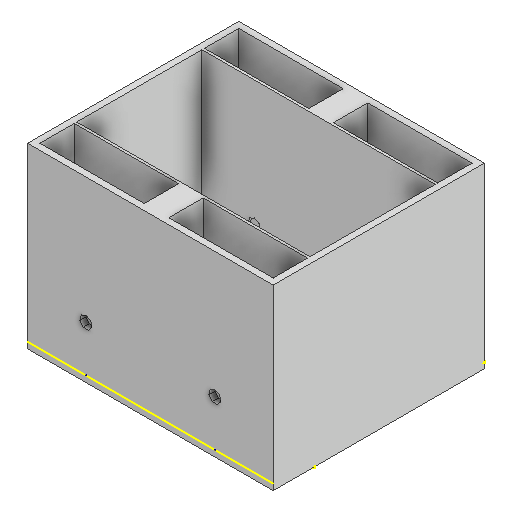
# Autodesk Inventor part: Part2
Saved by Autodesk Inventor 2026.2 (Build 302298010, 298A)
## iProperties
Created: 2026-05-07
Part Number: Part2
Material: Generic
Document SubType Name: Modeling
Designer: danie
Density: 1 g/cm^3
Appearance: Default
Author: danie
Autodesk Inventor part; units mm, degrees
ref_plane "YZ Plane" through (0, 0, 0) normal (1, 0, 0) x (0, 1, 0)
ref_plane "XZ Plane" through (0, 0, 0) normal (0, 1, 0) x (-1, 0, 0)
ref_plane "XY Plane" through (0, 0, 0) normal (0, 0, 1) x (1, 0, 0)
sketch "Sketch1" plane through (0, 0, 0) normal (0, 1, 0) x (-1, 0, 0)
  line L0 (0, 0) -> (200, 0)
  line L1 (200, 0) -> (200, 172)
  line L2 (200, 172) -> (0, 172)
  line L3 (0, 172) -> (0, 0)
  line L4 (0, 172) -> (200, 172)
  line L5 (200, 172) -> (200, -28)
  line L6 (200, -28) -> (0, -28)
  line L7 (0, -28) -> (0, 172)
  line L8 (200, 172) -> (195, 172)
  line L9 (195, 172) -> (195, 167)
  line L10 (195, 167) -> (200, 167)
  line L11 (195, 172) -> (195, 144)
  line L12 (195, 167) -> (130, 167)
  line L13 (130, 167) -> (130, 144)
  line L14 (130, 144) -> (195, 144)
  line L15 (195, 144) -> (195, 0)
  line L16 (195, 0) -> (195, 5)
  line L17 (195, 5) -> (130, 5)
  line L18 (130, 5) -> (130, 33)
  line L19 (130, 33) -> (195, 33)
  line L20 (0, 167) -> (5, 167)
  line L21 (5, 167) -> (5, 139)
  line L22 (130, 167) -> (130, 139)
  line L23 (130, 139) -> (195, 139)
  line L24 (5, 139) -> (70, 139)
  line L25 (70, 139) -> (70, 167)
  line L26 (70, 167) -> (5, 167)
  line L27 (5, 139) -> (5, 0)
  line L28 (5, 33) -> (70, 33)
  line L29 (70, 33) -> (70, 5)
  line L30 (70, 5) -> (5, 5)
  line L31 (130, 139) -> (70, 139)
  line L32 (130, 33) -> (70, 33)
  line L33 (130, 167) -> (70, 167)
  line L34 (130, 5) -> (70, 5)
  line L35 (37.5, 33) -> (37.5, 139)
  line L36 (162.5, 33) -> (162.5, 139)
  line L37 (5, 33) -> (7, 33)
  line L38 (5, 33) -> (5, 35)
  line L39 (5, 35) -> (195, 35)
  line L40 (195, 139) -> (197, 139)
  line L41 (5, 139) -> (5, 137)
  line L42 (5, 137) -> (195, 137)
  line L43 (100, 5) -> (90, 5)
  line L44 (90, 5) -> (110, 5)
  line L45 (110, 5) -> (110, 33)
  line L46 (90, 5) -> (90, 33)
  line L47 (90, 139) -> (90, 167)
  line L48 (110, 137) -> (110, 167)
  point P0 (110, 139)
  dimension "d0" = 200
  dimension "d1" = 172
  dimension "d2" = 200
  dimension "d3" = 200
  dimension "d4" = 5
  dimension "d5" = 5
  dimension "d6" = 28
  dimension "d7" = 65
  dimension "d8" = 5
  dimension "d9" = 28
  dimension "d10" = 5
  dimension "d11" = 28
  dimension "d12" = 28
  dimension "d13" = 65
  dimension "d14" = 2
  dimension "d15" = 2
  dimension "d16" = 2
  dimension "d17" = 2
  dimension "d18" = 10
  dimension "d19" = 20
  constraints: 98 end point, 36 point on line, 20 perpendicular, 6 parallel, 5 midpoint, 3 horizontal, 1 collinear
  measures "d0" distance of L2.end L1.end
  measures "d1" distance of L1.end L0.end
  measures "d2" distance of L5.end L6.end
  measures "d3" distance of L4.end L5.end
  measures "d4" distance of L4.end L8.end
  measures "d5" distance of L8.end L9.end
  measures "d6" distance of L8.end L11.end
  measures "d7" distance of L9.end L12.end
  measures "d8" distance of L15.end L16.end
  measures "d9" distance of L17.end L18.end
  measures "d10" distance of L20.start L20.end
  measures "d11" distance of L20.end L21.end
  measures "d12" distance of L12.end L22.end
  measures "d13" distance of L21.end L24.end
  measures "d14" distance of L28.start L37.end
  measures "d15" distance of L28.start L38.end
  measures "d16" distance of L23.end L40.end
  measures "d17" distance of L21.end L41.end
  measures "d18" distance of L43.start L43.end
  measures "d19" distance of L43.end L44.end
extrude "Extrusion1" add sketch "Sketch1" along normal blind 145 contours L3 L20 L21 L27 L0 | L27 L30 L34 L17 L15 L0 | L3 L2 L9 L12 L33 L26 L20 | L15 L11 L10 L1 L0 | L27 L39 L35 L28 | L2 L1 L10 L9 | L24 L35 L42 L27 | L19 L36 L39 L15 | L28 L35 L39 L36 L19 L32 | L46 L32 L45 L34 | L24 L31 L48 L42 L35 | L33 L48 L31 L47 | L42 L36 L23 L15 | L48 L31 L23 L36 L42
sketch "Sketch2" plane through (0, 0, 0) normal (0, -1, 0) x (1, 0, 0)
  line L0 (-5, 137) -> (-195, 137) projected
  line L1 (-195, 35) -> (-5, 35) projected
  line L2 (-195, 137) -> (-5, 137)
  line L3 (-5, 137) -> (-5, 35)
  line L4 (-5, 35) -> (-195, 35)
  line L5 (-195, 35) -> (-195, 137)
  point P0 (0, 0)
  constraints: 8 end point, 2 parallel, 1 horizontal, 1 perpendicular
extrude "Extrusion2" add sketch "Sketch2" against normal blind 5
sketch "Sketch3" plane through (-195, 0, 139) normal (0, 0, 1) x (1, 0, 0)
  point P0 (195, 0)
sketch "Sketch4" plane through (0, 5, 0) normal (0, 1, 0) x (1, 0, 0)
  line L0 (-90, -33) -> (-90, -5) projected
  line L1 (-5, -33) -> (-90, -33) projected
  line L2 (-90, -33) -> (-5, -33)
  line L3 (-5, -33) -> (-47.5, -33)
  line L4 (-47.5, -33) -> (-47.5, -172)
  line L5 (-200, -172) -> (0, -172) projected
  line L6 (-109.747, -33) -> (-194.7552, -33)
  line L7 (-194.7552, -33) -> (-109.747, -33)
  line L8 (-110, -5) -> (-110, -33) projected
  line L9 (-195, -5) -> (-110, -5) projected
  line L10 (-110, -5) -> (-195, -5)
  line L11 (-195, -5) -> (-152.5, -5)
  line L12 (-152.5, -5) -> (-152.5, -172)
  line L13 (-110, -167) -> (-195, -167) projected
  point P0 (0, 0)
  constraints: 16 end point, 3 collinear, 3 point on line, 2 midpoint, 2 perpendicular
sketch "Sketch5" plane through (-200, 0, 172) normal (0, 0, 1) x (1, 0, 0)
  line L0 (5, 144.4425) -> (89.9982, 145)
  line L1 (0, 145) -> (200, 145) projected
  line L2 (5, 144.4425) -> (47.1963, 145)
  line L3 (47.4991, 144.7212) -> (47.4991, 0)
  line L4 (0, 0) -> (200, 0) projected
  line L5 (200, 145) -> (195, 145)
  line L6 (195, 145) -> (110, 145)
  line L7 (110, 145) -> (152.5, 145)
  line L8 (152.5, 145) -> (152.5, 0)
  line L9 (195, 5) -> (5, 5) projected
  line L10 (152.5, 5) -> (152.5, 42.5)
  line L11 (152.5, 42.5) -> (47.4991, 42.5)
  circle A0 centre (47.4991, 42.5) radius 5
  circle A1 centre (152.5, 42.5) radius 5
  line L12 (47.4991, 47.5) -> (51.4082, 45.6174)
  line L13 (51.4082, 45.6174) -> (52.3737, 41.3874)
  line L14 (52.3737, 41.3874) -> (49.6685, 37.9952)
  line L15 (49.6685, 37.9952) -> (45.3297, 37.9952)
  line L16 (45.3297, 37.9952) -> (42.6244, 41.3874)
  line L17 (42.6244, 41.3874) -> (43.5899, 45.6174)
  line L18 (43.5899, 45.6174) -> (47.4991, 47.5)
  line L19 (152.5, 47.5) -> (156.4092, 45.6174)
  line L20 (156.4092, 45.6174) -> (157.3746, 41.3874)
  line L21 (157.3746, 41.3874) -> (154.6694, 37.9952)
  line L22 (154.6694, 37.9952) -> (150.3306, 37.9952)
  line L23 (150.3306, 37.9952) -> (147.6254, 41.3874)
  line L24 (147.6254, 41.3874) -> (148.5908, 45.6174)
  line L25 (148.5908, 45.6174) -> (152.5, 47.5)
  dimension "d29" = 10
  dimension "d30" = 10
  dimension "d24" = 85
  dimension "d25" = 42.2
  dimension "d26" = 5
  dimension "d27" = 85
  dimension "d28" = 37.5
  constraints: 46 end point, 11 point on line, 4 coincident, 2 midpoint, 2 perpendicular, 2 vertical alignment, 1 vertical, 34 other
  measures "d24" distance of L0.start L0.end
  measures "d25" distance of L0.start L2.end
  measures "d26" distance of L1.end L5.end
  measures "d27" distance of L5.end L6.end
  measures "d28" distance of L10.start L10.end
extrude "Extrusion3" cut sketch "Sketch5" against normal blind 376.75 contours L12 L13 L11 L3 | L3 L15 L16 L17 L18 | L11 L13 L14 L15 L3 | L19 L20 L21 L22 L8 | L8 L11 L24 L25 | L8 L22 L23 L24 L11
body "Solid1"
